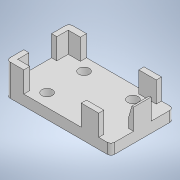
# Autodesk Inventor part: Крепление двигателя2
Saved by Autodesk Inventor 2020 (Build 240168000, 168)
## iProperties
Created: 2021-06-13
Part Number: Крепление двигателя2
Material: Типовые
Document SubType Name: Обычные детали
Designer: Антон
Density: 1 g/cm^3
Appearance: По умолчанию
Sheet Metal Rule: По умолчанию
Author: Антон
Autodesk Inventor part; units mm, degrees
ref_plane "YZ Plane" through (0, 0, 0) normal (1, 0, 0) x (0, 1, 0)
ref_plane "XZ Plane" through (0, 0, 0) normal (0, 1, 0) x (-1, 0, 0)
ref_plane "XY Plane" through (0, 0, 0) normal (0, 0, 1) x (1, 0, 0)
sketch "Эскиз1" plane through (0, 0, 0) normal (0, 1, 0) x (-1, 0, 0)
  line L0 (0, 0) -> (60, 0)
  line L1 (60, 0) -> (60, -36)
  line L2 (60, -36) -> (0, -36)
  line L3 (0, -36) -> (0, 0)
  dimension "d0" = 60
  dimension "d1" = 36
  constraints: 8 end point, 2 parallel, 1 horizontal, 1 perpendicular
  measures "d0" distance of L1.end L2.end
  measures "d1" distance of L0.end L1.end
extrude "Выдавливание1" add sketch "Эскиз1" along normal blind 6
sketch "Эскиз2" plane through (0, 6, 0) normal (0, 1, 0) x (1, 0, 0)
  line L0 (-60, 36) -> (-60, 0) projected
  line L1 (-60, 0) -> (0, 0) projected
  line L2 (-30, 0) -> (-30, 36)
  line L3 (0, 36) -> (-60, 36) projected
  line L4 (-60, 18) -> (0, 18)
  line L5 (0, 0) -> (0, 36) projected
  point P0 (-44, 7.4)
  point P1 (-44, 28.6)
  point P2 (-16, 7.4)
  point P3 (-16, 28.6)
  point P4 (-44, 7.4)
  dimension "d52" = 14
  dimension "d53" = 10.6
  constraints: 4 end point, 4 midpoint, 3 symmetric about line, 1 coincident
  measures "d52" distance from line of L2 point (-44, 7.4)
  measures "d53" distance from line of L4 point (-44, 7.4)
hole "Отверстие1" at (-44, 6, -7.4) at (-44, 6, -28.6) at (-16, 6, -28.6) at (-16, 6, -7.4) direction (0, -1, 0) diameter 3.2 end through all counterbore diameter 6 counterbore depth 5
sketch "Эскиз4" plane through (0, 0, -2.95) normal (1, 0, 0) x (0, 0, -1)
  line L0 (15.05, 0) -> (15.05, -13.5)
  circle A0 centre (15.05, -13.5) radius 18.5
  line L1 (-2.95, 3) -> (33.05, 3)
  line L2 (-2.95, 0) -> (-2.95, 6) projected
  line L3 (33.05, 0) -> (33.05, 6) projected
  line L4 (-2.95, 0) -> (33.05, 0) projected
  dimension "d27" = 13.5
  dimension "d38" = 37
  constraints: 4 end point, 3 midpoint, 1 centre point, 1 coincident, 1 vertical
  measures "d27" distance of L0.start L0.end
  measures "d38" diameter of A0
ref_plane "РабПлоскость3" through (-20, 0, 0) normal (1, 0, 0) x (0, 0, -1)
ref_plane "РабПлоскость2" through (-30, 0, 0) normal (1, 0, 0) x (0, 0, -1)
sketch "Эскиз13" plane through (0, 6, 0) normal (0, 1, 0) x (1, 0, 0)
  line L0 (0, 36) -> (-60, 36) projected
  line L1 (-60, 36) -> (-57, 36)
  line L2 (-57, 36) -> (-57, 26)
  line L3 (-57, 26) -> (-60, 26)
  line L4 (-60, 26) -> (-60, 36)
  line L5 (-60, 36) -> (-50, 36)
  line L6 (-50, 36) -> (-50, 32.5)
  line L7 (-50, 32.5) -> (-60, 32.5)
  line L8 (-60, 32.5) -> (-60, 36)
  line L9 (-60, 36) -> (-60, 0) construction
  line L10 (-60, 18) -> (0, 18) construction
  line L11 (0, 0) -> (0, 36) construction
  line L12 (-60, 0) -> (-57, 0)
  line L13 (-57, 0) -> (-57, 10)
  line L14 (-57, 10) -> (-60, 10)
  line L15 (-60, 10) -> (-60, 0)
  line L16 (-60, 0) -> (-50, 0)
  line L17 (-50, 0) -> (-50, 3.5)
  line L18 (-50, 3.5) -> (-60, 3.5)
  line L19 (-60, 3.5) -> (-60, 0)
  line L20 (0, 23) -> (-3, 23)
  line L21 (-3, 23) -> (-3, 13)
  line L22 (-3, 13) -> (0, 13)
  line L23 (0, 13) -> (0, 23)
  line L24 (-7, 36) -> (-17, 36)
  line L25 (-17, 36) -> (-17, 33)
  line L26 (-17, 33) -> (-7, 33)
  line L27 (-7, 33) -> (-7, 36)
  line L28 (-7, 0) -> (-17, 0)
  line L29 (-17, 0) -> (-17, 3)
  line L30 (-17, 3) -> (-7, 3)
  line L31 (-7, 3) -> (-7, 0)
  line L32 (-60, 0) -> (0, 0) projected
  point P0 (-57, 32.5)
  point P1 (-57, 3.5)
  point P2 (-17, 34.5)
  point P3 (-17, 1.5)
  dimension "d88" = 3
  dimension "d89" = 3.5
  dimension "d90" = 10
  dimension "d93" = 10
  dimension "d97" = 7
  constraints: 58 end point, 10 parallel, 6 equal length, 6 midpoint, 6 symmetric about line, 5 horizontal, 5 perpendicular, 2 collinear, 1 vertical alignment
  measures "d88" distance of L2.end L3.end
  measures "d89" distance of L5.end L6.end
  measures "d90" distance of L1.end L2.end
  measures "d93" distance of L20.end L21.end
  measures "d97" distance between parallel lines of L11 L27
extrude "Выдавливание8" add sketch "Эскиз13" along normal blind 12
chamfer "Фаска1" distance 2 distance2 7 1 edges at (-3, 18, -18) measured on face at (-2.5, 18, -18)
extrude "Выдавливание3" cut sketch "Эскиз4" against normal blind 7 from surface at -20 contours A0 L4 | L4 A0 L1 | L1 A0
fillet "Сопряжение3" radius 2.15 4 edges at (-60, 9, 0) (-60, 9, -36) (0, 3, 0) (0, 3, -36)
equation "\"Радиус_гибки\" = Толщина"
equation "\"Ширина_просечки\" = Толщина"
equation "\"Глубина_просечки\" = 0.5 * Толщина"
equation "\"Размер_просечки\" = 4 * Толщина"
equation "\"Мин_остаток\" = 2 * Толщина"
equation "\"Радиус_перехода\" = Радиус_гибки"
equation "\"Радиус_Якоби\" = Толщина"
equation "\"Размер_зазора\" = Толщина"
equation "\"Толщина\" = 0.5"
